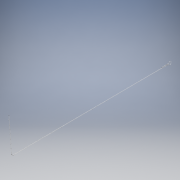
# Autodesk Inventor part: +XPanel_AntennaString
Saved by Autodesk Inventor 2018 (Build 220112000, 112)
## iProperties
Created: 2018-10-31
Part Number: +XPanel_AntennaString
Material: Acrylic, Clear
Document SubType Name: Modeling
Designer: Bradley
Density: 1.19 g/cm^3
Appearance: Transparent - Clear
Author: Bradley
Autodesk Inventor part; units mm, degrees
ref_plane "YZ Plane" through (0, 0, 0) normal (1, 0, 0) x (0, 1, 0)
ref_plane "XY Plane" through (0, 0, 0) normal (0, 0, 1) x (1, 0, 0)
sketch "Sketch2" plane through (0, 0, 0) normal (1, 0, 0) x (0, 1, 0)
  circle A0 centre (-29.5, 0) radius 0.4 construction
  circle A1 centre (29.5, 0) radius 0.4 construction
  line L0 (-29.5, 0) -> (29.5, 0) construction
  line L1 (-31.024, 13.15) -> (-29.9985, -0.0388)
  arc A2 (-29.9985, -0.0388) -> (-29.4966, -0.5) centre (-29.5, 0) ccw
  line L2 (-29.4966, -0.5) -> (28.4809, -0.1069)
  arc A3 (29.1626, -0.369) -> (28.4809, -0.1069) centre (28.4877, -1.1069) ccw
  arc A4 (29.1626, -0.369) -> (29.1576, 0.3644) centre (29.5, 0) ccw
  arc A5 (28.4795, 0.0931) -> (29.1576, 0.3644) centre (28.4728, 1.0931) ccw
  line L3 (28.4795, 0.0931) -> (26.4796, 0.0795)
  circle A6 centre (29.1626, -0.369) radius 0.1 construction
  line L4 (28.4795, 0.0931) -> (28.4809, -0.1069) construction
  line L5 (28.4802, -0.0069) -> (29.5, 0) construction
  point P0 (0, 0)
  point P1 (0, 0)
  dimension "d5" = 0.8
  dimension "d6" = 59
  dimension "d7" = 0.2
  dimension "d8" = 0.2
  dimension "d9" = 1
  dimension "d10" = 2
  dimension "d11" = 1.524
  dimension "d12" = 13.15
  constraints: 12 end point, 8 point on circle, 7 centre point, 7 tangent, 4 coincident, 3 equal radius, 2 midpoint, 1 horizontal, 1 parallel, 1 perpendicular
  measures "d5" diameter of A0
  measures "d6" distance of L0.start L0.end
  measures "d7" diameter of A6
  measures "d8" distance between parallel lines of L2 L3
  measures "d9" radius of A5
  measures "d10" distance of L3.start L3.end
  measures "d11" horizontal distance of L0.start L1.start
  measures "d12" vertical distance of L0.start L1.start
ref_plane "Work Plane1" through (0, 29.5, 0) normal (0, 1, 0) x (-1, 0, 0)
sketch "Sketch3" plane through (0, 29.5, 0) normal (0, 1, 0) x (-1, 0, 0)
  line L0 (0, 0.5) -> (0, -0.5) projected
  circle A0 centre (0, -0.5) radius 0.1
  point P0 (0, 0)
  point P1 (0, -0.369)
  point P2 (0, 0.3644)
  dimension "d13" = 0.2
  constraints: 1 centre point, 1 coincident
  measures "d13" diameter of A0
sweep "Sweep1" add profiles "Sketch3" path "Sketch2"
equation "\"d8\" = d7"
equation "\"d13\" = d7"
body "Solid1"
